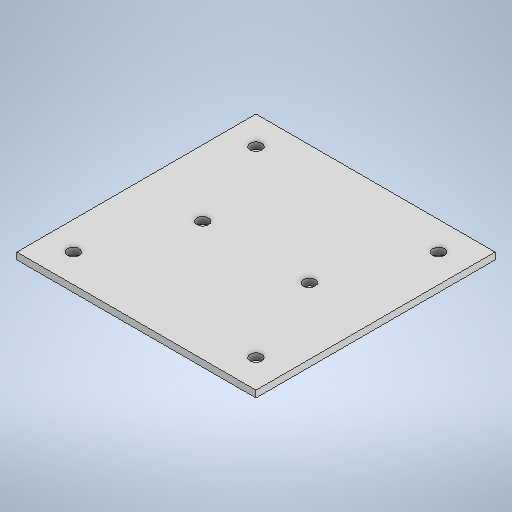
# Autodesk Inventor part: DIFF_HOUSING_TOP
Saved by Autodesk Inventor 2025.1 (Build 291241000, 241)
## iProperties
Created: 2023-11-30
Part Number: DIFF_HOUSING_TOP
Material: Generic
Document SubType Name: Modeling
Designer: bugme
Density: 1 g/cm^3
Appearance: Default
Author: bugme
Autodesk Inventor part; units mm, degrees
ref_plane "YZ Plane" through (0, 0, 0) normal (1, 0, 0) x (0, 1, 0)
ref_plane "XZ Plane" through (0, 0, 0) normal (0, 1, 0) x (-1, 0, 0)
ref_plane "XY Plane" through (0, 0, 0) normal (0, 0, 1) x (1, 0, 0)
sketch "Sketch1" plane through (0, 0, 0) normal (0, 1, 0) x (-1, 0, 0)
  line L0 (55.88, 55.88) -> (-55.88, 55.88)
  line L1 (-55.88, 55.88) -> (-55.88, -55.88)
  line L2 (-55.88, -55.88) -> (55.88, -55.88)
  line L3 (55.88, -55.88) -> (55.88, 55.88)
  line L4 (78.232, 0) -> (-78.232, 0) projected
  line L5 (0, -78.232) -> (0, 78.232) projected
  point P0 (0, 0)
  dimension "d0" = 111.76
  dimension "d1" = 111.76
  constraints: 8 end point, 2 parallel, 2 symmetric about line, 1 horizontal, 1 perpendicular
  measures "d0" distance of L2.end L1.end
  measures "d1" distance of L0.end L1.end
extrude "Extrusion1" add sketch "Sketch1" along normal blind 3.175
sketch "Sketch2" plane through (0, 3.175, 0) normal (0, 1, 0) x (1, 0, 0)
  line L0 (-55.88, 55.88) -> (-55.88, -55.88) projected
  line L1 (-55.88, -55.88) -> (-55.88, -42.705)
  line L2 (-55.88, -42.705) -> (-42.705, -42.705)
  point P0 (0, 0)
  dimension "d4" = 13.175
  dimension "d5" = 13.175
  constraints: 4 end point, 1 perpendicular, 1 point on line
  measures "d4" distance of L0.end L1.end
  measures "d5" distance of L1.end L2.end
hole "Hole1" at (-42.705, 3.175, 42.705) direction (0, -1, 0) diameter 5.5118 depth 14.1986 tip angle 118 clearance for "Flat Head Machine Screw" size "M5" standard "Ansi Metric M Profile"
mirror "Mirror4" about plane through (0, 0, 0) normal (0, 0, 1) of "Hole1"
mirror "Mirror5" about plane through (0, 0, 0) normal (1, 0, 0) of "Hole1", "Mirror4"
sketch "Sketch4" plane through (0, 3.175, 0) normal (0, 1, 0) x (1, 0, 0)
  line L0 (-55.88, -55.88) -> (55.88, -55.88) projected
  line L1 (-78.232, 0) -> (78.232, 0) projected
  line L2 (55.88, -55.88) -> (55.88, 55.88) projected
  line L3 (-55.88, 55.88) -> (-55.88, -55.88) projected
  point P0 (0, 0)
  point P1 (24.892, 0)
  point P2 (-24.892, 0)
  dimension "d26" = 30.988
  dimension "d27" = 30.988
  constraints: 2 point on line
  measures "d26" distance from line of L2 point (24.892, 0)
  measures "d27" distance from line of L3 point (-24.892, 0)
hole "Hole2" at (24.892, 3.175, 0) at (-24.892, 3.175, 0) direction (0, -1, 0) diameter 5.5118 end through all clearance for "Flat Head Machine Screw" size "M5" standard "Ansi Metric M Profile"
equation "\"d0\" = d1"
equation "\"d4\" = d5"
body "Solid1"
